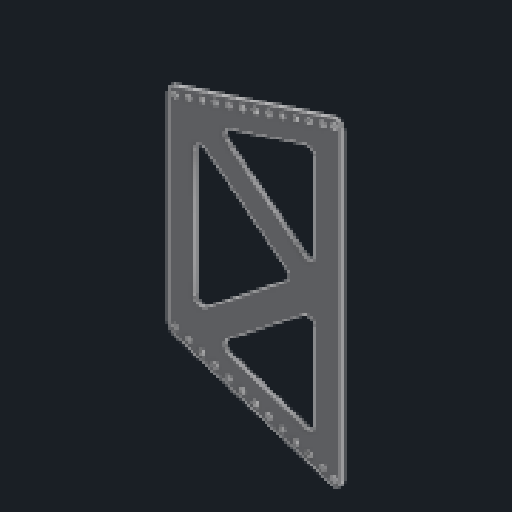
# Autodesk Inventor part: Part1
Saved by Autodesk Inventor 2025.2 (Build 292293000, 293)
## iProperties
Created: 2025-09-26
Part Number: Part1
Material: Generic
Document SubType Name: Sheet Metal
Designer: valer
Density: 1 g/cm^3
Sheet Metal Rule: Default
Appearance: Default
Author: valer
Autodesk Inventor part; units mm, degrees
ref_plane "YZ Plane" through (0, 0, 0) normal (1, 0, 0) x (0, 1, 0)
ref_plane "XZ Plane" through (0, 0, 0) normal (0, 1, 0) x (-1, 0, 0)
ref_plane "XY Plane" through (0, 0, 0) normal (0, 0, 1) x (1, 0, 0)
sketch "Base" plane through (0, 0, 0) normal (0, 0, 1) x (1, 0, 0)
  line L0 (-173.8499, -66.2658) -> (171.6188, -178.9186) construction
  line L1 (-9.525, -101.5493) -> (-9.525, 101.5493) construction
  line L2 (-9.525, 0) -> (-9.525, -119.85)
  line L3 (187.0398, -183.9472) -> (-9.525, -119.85)
  line L4 (187.0398, -183.9472) -> (187.0398, 0)
  line L5 (187.0398, 0) -> (-9.525, 0) construction
  line L6 (-9.525, 0) -> (-9.525, 119.85)
  line L7 (187.0398, 183.9472) -> (-9.525, 119.85)
  line L8 (187.0398, 183.9472) -> (187.0398, 0)
  point P0 (0, 0)
  point P1 (187.0398, -182.4643)
extrude "Plate1" add sketch "Base" along normal blind 3.048
fillet "OutsideFilletsFeature" radius 8 4 edges at (187.0398, 183.9472, 1.524) (187.0398, -183.9472, 1.524) (-9.525, 119.85, 1.524) (-9.525, -119.85, 1.524)
sketch "MountHoles" plane through (0, 0, 0) normal (0, 0, -1) x (-1, 0, 0)
  arc A0 (-176.5597, 180.5298) -> (-187.0398, 172.9239) centre (-179.0398, 172.9239) ccw projected
  arc A1 (9.525, 114.0441) -> (4.0052, 121.6499) centre (1.525, 114.0441) ccw projected
  line L0 (-179.0398, 172.9239) -> (1.525, 114.0441) construction
  circle A2 centre (-179.0398, 172.9239) radius 3
  circle A3 centre (1.525, 114.0441) radius 3
  line L1 (-228.9265, 0) -> (50.7072, 0) construction
  circle A4 centre (-179.0398, -172.9239) radius 3
  circle A5 centre (1.525, -114.0441) radius 3
  circle A6 centre (-13.6867, 119.0044) radius 3
  circle A7 centre (-28.8984, 123.9648) radius 3
  circle A8 centre (-44.11, 128.9251) radius 3
  circle A9 centre (-59.3217, 133.8854) radius 3
  circle A10 centre (-74.5334, 138.8457) radius 3
  circle A11 centre (-89.7451, 143.8061) radius 3
  circle A12 centre (-104.9567, 148.7664) radius 3
  circle A13 centre (-120.1684, 153.7267) radius 3
  circle A14 centre (-135.3801, 158.6871) radius 3
  circle A15 centre (-150.5918, 163.6474) radius 3
  circle A16 centre (-165.8035, 168.6077) radius 3
  circle A17 centre (-13.6867, -119.0044) radius 3
  circle A18 centre (-28.8984, -123.9648) radius 3
  circle A19 centre (-44.11, -128.9251) radius 3
  circle A20 centre (-59.3217, -133.8854) radius 3
  circle A21 centre (-74.5334, -138.8457) radius 3
  circle A22 centre (-89.7451, -143.8061) radius 3
  circle A23 centre (-104.9567, -148.7664) radius 3
  circle A24 centre (-120.1684, -153.7267) radius 3
  circle A25 centre (-135.3801, -158.6871) radius 3
  circle A26 centre (-150.5918, -163.6474) radius 3
  circle A27 centre (-165.8035, -168.6077) radius 3
  point P0 (0, 0)
  dimension "d2" = 6
  dimension "d3" = 6
  dimension "d28" = 16
  constraints: 26 centre point, 13 symmetric about line, 2 coincident, 2 end point, 36 other
  measures "d2" diameter of A2
  measures "d3" diameter of A3
  measures "d28" distance of A3.centre A6.centre
extrude "MountHolesFeature" cut sketch "MountHoles" against normal blind 3.048
sketch "MiddleCuts" plane through (0, 0, 3.048) normal (0, 0, 1) x (1, 0, 0)
  line L0 (20.475, -87.6609) -> (132.6758, 0)
  line L1 (132.6758, 0) -> (20.475, 87.6609)
  line L2 (20.475, 87.6609) -> (20.475, -87.6609)
  line L3 (157.0398, 19.0353) -> (45.4472, 106.221)
  line L4 (45.4472, 106.221) -> (157.0398, 142.6099)
  line L5 (157.0398, 142.6099) -> (157.0398, 19.0353)
  line L6 (-48.838, 0) -> (226.3528, 0) construction
  line L7 (-9.525, -114.0441) -> (-9.525, 114.0441) projected
  line L8 (-4.0052, 121.6499) -> (176.5597, 180.5298) projected
  line L9 (187.0398, 172.9239) -> (187.0398, -172.9239) projected
  line L10 (157.0398, -19.0353) -> (45.4472, -106.221)
  line L11 (45.4472, -106.221) -> (157.0398, -142.6099)
  line L12 (157.0398, -142.6099) -> (157.0398, -19.0353)
  point P0 (0, 0)
  dimension "d18" = 30
  dimension "d19" = 30
  dimension "d20" = 30
  dimension "d21" = 30
  dimension "d22" = 38
  constraints: 18 end point, 4 parallel, 3 symmetric about line, 2 point on line, 1 equal length, 1 perpendicular
  measures "d18" distance between parallel lines of L7 L2
  measures "d19" distance between parallel lines of L8 L4
  measures "d20" distance between parallel lines of L3 L1
  measures "d21" distance between parallel lines of L9 L5
  measures "d22" angle of L1 L6
extrude "MiddleCutsFeature" cut sketch "MiddleCuts" against normal blind 3.048
fillet "InsideFilletsFeature" radius 8 9 edges at (20.475, -87.6609, 1.524) (20.475, 87.6609, 1.524) (45.4472, 106.221, 1.524) (45.4472, -106.221, 1.524) (157.0398, -142.6099, 1.524) (157.0398, -19.0353, 1.524) (132.6758, 0, 1.524) (157.0398, 19.0353, 1.524) (157.0398, 142.6099, 1.524)
equation "\"d7\" = Thickness"
equation "\"d19\" = d18"
equation "\"d23\" = Thickness"
equation "\"d0\" = Thickness"
equation "\"BendRadius\" = Thickness"
equation "\"BendReliefWidth\" = Thickness"
equation "\"BendReliefDepth\" = 0.5 * Thickness"
equation "\"CornerReliefSize\" = 4 * Thickness"
equation "\"MinimumRemnant\" = 2 * Thickness"
equation "\"TransitionRadius\" = BendRadius"
equation "\"JacobiRadiusSize\" = BendRadius"
equation "\"GapSize\" = Thickness"
equation "\"Thickness\" = 3.048"
body "Solid1"
